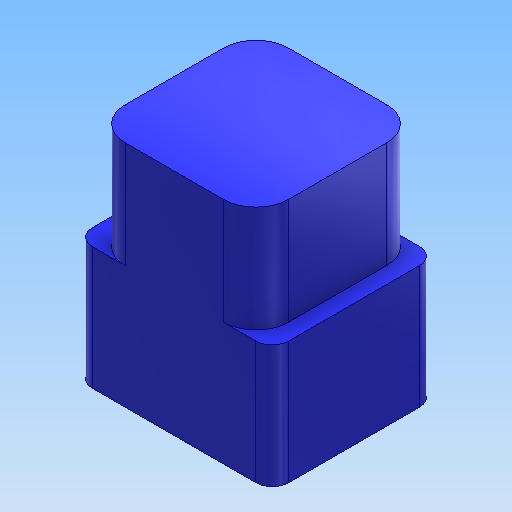
# Autodesk Inventor part: Taster
Saved by Autodesk Inventor 2018 (Build 220112000, 112)
## iProperties
Created: 2020-10-03
Part Number: Taster
Material: Generisch
Document SubType Name: Modeling
Designer: marce
Density: 1 g/cm^3
Appearance: Blau - Wandfarbe - glänzend
Author: marce
Autodesk Inventor part; units mm, degrees
ref_plane "YZ Plane" through (0, 0, 0) normal (1, 0, 0) x (0, 1, 0)
ref_plane "XZ Plane" through (0, 0, 0) normal (0, 1, 0) x (-1, 0, 0)
ref_plane "XY Plane" through (0, 0, 0) normal (0, 0, 1) x (1, 0, 0)
sketch "Skizze1" plane through (0, 0, 0) normal (0, 0, 1) x (1, 0, 0)
  line L0 (0, 0) -> (12, 0)
  line L1 (12, 0) -> (12, 10)
  line L2 (12, 10) -> (0, 10)
  line L3 (0, 10) -> (0, 0)
  dimension "d0" = 12
  dimension "d1" = 10
  constraints: 8 end point, 2 parallel, 1 horizontal, 1 perpendicular
  measures "d0" distance of L2.end L1.end
  measures "d1" distance of L1.end L0.end
extrude "Extrusion1" add sketch "Skizze1" along normal blind 14
sketch "Skizze2" plane through (0, 0, 14) normal (0, 0, 1) x (1, 0, 0)
  line L0 (1, 10) -> (11, 10)
  line L1 (11, 10) -> (11, 0)
  line L2 (11, 0) -> (1, 0)
  line L3 (1, 0) -> (1, 10)
  line L4 (12, 10) -> (0, 10) projected
  line L5 (0, 10) -> (0, 0) projected
  line L6 (0, 0) -> (12, 0) projected
  line L7 (0, 10) -> (12, 10)
  line L8 (12, 10) -> (12, 0)
  line L9 (12, 0) -> (0, 0)
  line L10 (0, 0) -> (0, 10)
  point P0 (6, 10)
  point P1 (6, 10)
  point P2 (1, 5)
  point P3 (0, 5)
  dimension "d4" = 10
  dimension "d5" = 10
  constraints: 16 end point, 4 midpoint, 4 parallel, 2 horizontal, 2 perpendicular, 1 coincident, 1 horizontal alignment
  measures "d4" distance of L1.end L2.end
  measures "d5" distance of L0.end L1.end
extrude "Extrusion2" cut sketch "Skizze2" against normal blind 6.5 contours L3 L6 L5 L4 | L4 L8 L6 L1
fillet "Rundung1" radius 2 4 edges at (11, 0, 10.75) (11, 10, 10.75) (1, 0, 10.75) (1, 10, 10.75)
fillet "Rundung2" radius 1 4 edges at (0, 0, 3.75) (0, 10, 3.75) (12, 0, 3.75) (12, 10, 3.75)
